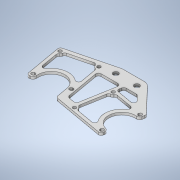
# Autodesk Inventor part: Knee_side_frame
Saved by Autodesk Inventor 2020.4 (Build 244396000, 396)
## iProperties
Created: 2021-09-05
Part Number: Knee_side_frame
Material: アルミニウム 2014-T4
Document SubType Name: Modeling
Designer: Masato Kubotera
Density: 2.8 g/cm^3
Appearance: 滑らか - 淡い灰色
Mass: 7.94371 g
Surface Area: 42.7962 cm^2
Volume: 2.83704 cm^3
Description: A2017 T2
Author: Masato Kubotera
Autodesk Inventor part; units mm, degrees
ref_plane "YZ Plane" through (0, 0, 0) normal (1, 0, 0) x (0, 1, 0)
ref_plane "XZ Plane" through (0, 0, 0) normal (0, 1, 0) x (-1, 0, 0)
ref_plane "XY Plane" through (0, 0, 0) normal (0, 0, 1) x (1, 0, 0)
sketch "スケッチ1" plane through (0, 0, 0) normal (0, 0, 1) x (1, 0, 0)
  line L0 (-46.5961, 42.1731) -> (-4.2493, 49.64) construction
  line L1 (-4.2493, 49.64) -> (1.3074, 18.1262) construction
  line L2 (1.3074, 18.1262) -> (-41.0393, 10.6593) construction
  line L3 (-41.0393, 10.6593) -> (-46.5961, 42.1731) construction
  line L4 (-46.5961, 42.1731) -> (1.3074, 18.1262) construction
  line L5 (-4.2493, 49.64) -> (-41.0393, 10.6593) construction
  line L6 (-43.8177, 26.4162) -> (-1.471, 33.8831) construction
  line L7 (-6.7696, 46.6571) -> (-33.3594, 41.9686) construction
  line L8 (-33.3594, 41.9686) -> (-28.6709, 15.3787) construction
  line L9 (-28.6709, 15.3787) -> (-2.0811, 20.0672) construction
  line L10 (-2.0811, 20.0672) -> (-6.7696, 46.6571) construction
  line L11 (-6.7696, 46.6571) -> (-28.6709, 15.3787) construction
  line L12 (-33.3594, 41.9686) -> (-2.0811, 20.0672) construction
  circle A0 centre (-32, 28.5) radius 10.5 construction
  line L13 (-20.0645, 44.3128) -> (-15.376, 17.723) construction
  circle A1 centre (-6.7696, 46.6571) radius 1.35
  circle A2 centre (-2.0811, 20.0672) radius 1.35
  arc A3 (-36.1041, 41.4846) -> (-33.0796, 39.1957) centre (-33.3594, 41.9686) ccw
  line L14 (-36.1041, 41.4846) -> (-36.5382, 43.9466)
  circle A4 centre (0, 8.5) radius 2.05
  circle A5 centre (0, 8.5) radius 6 construction
  circle A6 centre (0, 8.5) radius 4.6 construction
  line L15 (-36.5382, 43.9466) -> (-4.2493, 49.64)
  line L16 (-4.2493, 49.64) -> (5.8157, 9.9758)
  arc A7 (6, 8.5) -> (5.8157, 9.9758) centre (0, 8.5) ccw
  circle A8 centre (-32, -28.5) radius 10.5 construction
  line L17 (-31.7738, 42.2481) -> (-9.2317, 46.2229)
  arc A9 (-27.0853, 15.6583) -> (-31.7738, 42.2481) centre (-32, 28.5) ccw
  line L18 (-27.0853, 15.6583) -> (-4.5432, 19.6331)
  line L19 (-5.9851, 44.2833) -> (-0.2802, 21.8012)
  arc A10 (-9.2317, 46.2229) -> (-5.9851, 44.2833) centre (-6.7696, 46.6571) ccw
  arc A11 (-0.2802, 21.8012) -> (-4.5432, 19.6331) centre (-2.0811, 20.0672) ccw
  arc A12 (-32.03, 42.203) -> (-34.6889, 41.7341) centre (-33.3594, 41.9686) ccw
  arc A13 (-34.6021, 41.2417) -> (-31.9431, 41.7106) centre (-33.2726, 41.4761) ccw
  line L20 (-34.6889, 41.7341) -> (-34.6021, 41.2417)
  line L21 (-31.9431, 41.7106) -> (-32.03, 42.203)
  arc A14 (-30.0004, 15.1443) -> (-27.3415, 15.6132) centre (-28.6709, 15.3787) ccw
  arc A15 (-27.4283, 16.1056) -> (-30.0873, 15.6367) centre (-28.7578, 15.8711) ccw
  line L22 (-30.0004, 15.1443) -> (-30.0873, 15.6367)
  line L23 (-27.4283, 16.1056) -> (-27.3415, 15.6132)
  line L24 (-49.8407, -37.5393) -> (-42.3738, 4.8074) construction
  line L25 (-42.3738, 4.8074) -> (-10.86, -0.7493) construction
  line L26 (-10.86, -0.7493) -> (-18.3269, -43.0961) construction
  line L27 (-18.3269, -43.0961) -> (-49.8407, -37.5393) construction
  line L28 (-49.8407, -37.5393) -> (-10.86, -0.7493) construction
  line L29 (-42.3738, 4.8074) -> (-18.3269, -43.0961) construction
  line L30 (-34.0838, -40.3177) -> (-26.6169, 2.029) construction
  line L31 (-18.5314, -29.8594) -> (-13.8429, -3.2696) construction
  line L32 (-13.8429, -3.2696) -> (-40.4328, 1.4189) construction
  line L33 (-40.4328, 1.4189) -> (-45.1213, -25.1709) construction
  line L34 (-45.1213, -25.1709) -> (-18.5314, -29.8594) construction
  line L35 (-18.5314, -29.8594) -> (-40.4328, 1.4189) construction
  line L36 (-13.8429, -3.2696) -> (-45.1213, -25.1709) construction
  circle A16 centre (-40.4328, 1.4189) radius 1.35
  arc A17 (-44.8868, -23.8415) -> (-45.3557, -26.5004) centre (-45.1213, -25.1709) ccw
  line L37 (-44.8868, -23.8415) -> (-44.3944, -23.9283)
  line L38 (-44.8633, -26.5873) -> (-45.3557, -26.5004)
  arc A18 (-44.8633, -26.5873) -> (-44.3944, -23.9283) centre (-44.6289, -25.2578) ccw
  line L39 (-32, -28.5) -> (-32, 28.5) construction
  line L40 (-13.8429, -3.2696) -> (-18.5314, -29.8594) construction
  circle A19 centre (-13.8429, -3.2696) radius 1.35
  arc A20 (-18.7659, -31.1889) -> (-18.297, -28.53) centre (-18.5314, -29.8594) ccw
  line L41 (-18.297, -28.53) -> (-18.7894, -28.4431)
  line L42 (-19.2583, -31.1021) -> (-18.7659, -31.1889)
  arc A21 (-18.7894, -28.4431) -> (-19.2583, -31.1021) centre (-19.0239, -29.7726) ccw
  circle A22 centre (0, -8.5) radius 2.05
  circle A23 centre (0, -8.5) radius 6 construction
  line L43 (0, 8.5) -> (0, -8.5) construction
  arc A24 (-30.1333, 17.9133) -> (-33.0796, 39.1957) centre (-32, 28.5) ccw
  arc A25 (-21.3013, -29.5493) -> (-42.4123, -25.8268) centre (-32, -28.5) ccw
  arc A26 (-20.4814, -20.991) -> (-40.2557, -17.5043) centre (-32, -28.5) ccw
  line L44 (-47.9807, -26.9905) -> (-45.0262, -27.5114)
  arc A27 (-45.0262, -27.5114) -> (-42.4123, -25.8268) centre (-44.6289, -25.2578) ccw
  arc A28 (-21.3013, -29.5493) -> (-19.4212, -32.0263) centre (-19.0239, -29.7726) ccw
  line L45 (-16.4668, -32.5472) -> (4.1466, -12.8365)
  line L46 (6, -8.5) -> (6, 8.5)
  arc A29 (4.1466, -12.8365) -> (6, -8.5) centre (0, -8.5) ccw
  line L47 (-14.8529, -23.3942) -> (-6, -14.929)
  arc A30 (-40.8669, -1.0432) -> (-37.9337, 1.4859) centre (-40.4328, 1.4189) ccw
  line L48 (-43.4262, -15.5576) -> (-40.8669, -1.0432)
  line L49 (-37.9337, 1.4859) -> (-16.1684, -2.3519)
  arc A31 (-16.1684, -2.3519) -> (-14.2771, -5.7317) centre (-13.8429, -3.2696) ccw
  line L50 (-16.8364, -20.2461) -> (-14.2771, -5.7317)
  line L51 (-11.3809, -3.7038) -> (-14.8529, -23.3942)
  circle A32 centre (-13.8429, -3.2696) radius 2.4 construction
  arc A33 (-41.98, 15.994) -> (-29.2216, 12.7431) centre (-32, 28.5) ccw construction
  line L52 (-40.7981, 4.5296) -> (-39.3221, 12.9004) construction
  line L53 (-39.3221, 12.9004) -> (-10.9597, 7.8994) construction
  line L54 (-12.4357, -0.4715) -> (-10.9597, 7.8994) construction
  line L55 (-19.4212, -32.0263) -> (-16.4668, -32.5472)
  line L56 (-47.9807, -26.9905) -> (-40.3815, 16.1063)
  line L57 (-40.3815, 16.1063) -> (-30.1333, 17.9133)
  arc A34 (-11.3809, -3.7038) -> (-11.3438, -3.2026) centre (-13.8429, -3.2696) ccw
  line L58 (-11.3438, -3.2026) -> (-6, -4.1448)
  line L59 (-35.5876, 11.6206) -> (-36.9574, 3.8523)
  line L60 (-36.9574, 3.8523) -> (-6, -1.6063)
  line L61 (-6, -1.6063) -> (-6, 16.8377)
  line L62 (-35.5876, 11.6206) -> (-6, 16.8377)
  arc A35 (-43.4262, -15.5576) -> (-40.2557, -17.5043) centre (-41.4566, -15.9049) ccw
  arc A36 (-20.4814, -20.991) -> (-16.8364, -20.2461) centre (-18.806, -19.8988) ccw
  line L63 (-6, -4.1448) -> (-6, -14.929)
  point P0 (-22.6443, 30.1497)
  point P1 (-17.7203, 31.0179)
  point P2 (-30.3503, -19.1443)
  point P3 (-29.4821, -14.2203)
  point P4 (-29.4821, -14.2203)
  point P5 (-44.8417, -23.5853)
  point P6 (-18.2519, -28.2738)
  point P7 (31.7198, -6.6988)
  point P8 (-13.0711, -52.3219)
  point P9 (-12.9341, -52.334)
  point P10 (13.7499, -57.0391)
  point P11 (13.8829, -57.0746)
  point P12 (0, 0)
  point P13 (0, 0)
  dimension "d21" = 43
  dimension "d22" = 32
  dimension "d23" = 27
  dimension "d24" = 27
  dimension "d27" = 21
  dimension "d28" = 9.5
  dimension "d31" = 4.1
  dimension "d34" = 12
  dimension "d39" = 8.5
  dimension "d40" = 9.2
  dimension "d41" = 32
  dimension "d46" = 20
  dimension "d56" = 2.5
  dimension "d57" = 2.5
  dimension "d62" = 3
  dimension "d63" = 2.5
  dimension "d67" = 2.7
  dimension "d68" = 1.35
  dimension "d70" = 0.5
  dimension "d72" = 43
  dimension "d73" = 32
  dimension "d77" = 9.5
  dimension "d78" = 20
  dimension "d80" = 27
  dimension "d81" = 27
  dimension "d82" = 8.5
  dimension "d83" = 2.7
  dimension "d86" = 0.5
  dimension "d87" = 1.35
  dimension "d88" = 57
  dimension "d89" = 80
  dimension "d90" = 21
  dimension "d91" = 100
  dimension "d92" = 4.1
  dimension "d93" = 12
  dimension "d94" = 17
  dimension "d95" = 3
  dimension "d96" = 0.25
  dimension "d97" = 0.25
  dimension "d98" = 3
  dimension "d99" = 0
  dimension "d101" = 2.5
  dimension "d102" = 5.5
  dimension "d107" = 2.5
  dimension "d109" = 2.5
  dimension "d111" = 4.8
  dimension "d112" = 8.5
  dimension "d113" = 28.8
  dimension "d114" = 2.5
  dimension "d115" = 2.5
  dimension "d116" = 2
  dimension "d117" = 2
  dimension "d118" = 2.5
  dimension "d119" = 5.5
  dimension "d120" = 2.5
  constraints: 128 end point, 56 point on circle, 37 centre point, 24 coincident, 23 tangent, 22 parallel, 22 symmetric about line, 16 midpoint, 16 point on line, 11 perpendicular, 3 vertical, 2 collinear, 8 other
  measures "d21" distance of L1.end L2.end
  measures "d22" distance of L0.end L1.end
  measures "d23" distance of L9.end L8.end
  measures "d24" distance of L8.end L7.end
  measures "d27" diameter of A0
  measures "d28" distance of point (-22.644, 30.15) A0.centre
  measures "d31" diameter of A4
  measures "d34" diameter of A5
  measures "d39" distance from line of L8 point (-22.644, 30.15)
  measures "d40" diameter of A6
  measures "d41" horizontal distance of A4.centre A0.centre
  measures "d46" vertical distance of L43.start A0.centre
  measures "d56" radius of A10
  measures "d57" distance from line of L17.end L15
  measures "d62" distance between parallel lines of L16 L19
  measures "d63" radius of A11
  measures "d67" diameter of A1
  measures "d68" radius of A12
  measures "d70" distance of L21.start L21.end
  measures "d72" distance of L25.end L26.end
  measures "d73" distance of L24.end L25.end
  measures "d77" distance of L39.start point (-30.35, -19.144)
  measures "d78" angle of L25 L2
  measures "d80" distance of L31.start L31.end
  measures "d81" distance of L31.end L32.end
  measures "d82" distance from line of L34 point (-30.35, -19.144)
  measures "d83" diameter of A16
  measures "d86" distance of L33.end A18.centre
  measures "d87" radius of A17
  measures "d88" distance of L39.start A0.centre
  measures "d89" angle of L39 L2
  measures "d90" diameter of A8
  measures "d91" angle of L25 L39
  measures "d92" diameter of A22
  measures "d93" diameter of A23
  measures "d94" distance of L43.start L43.end
  measures "d95" radial gap between concentric circles of A24 A9
  measures "d96" radial gap between concentric circles of A0 A24
  measures "d97" radial gap between concentric circles of A8 A25
  measures "d98" radial gap between concentric circles of A25 A26
  measures "d99" distance between parallel lines of L9 L18
  measures "d101" radius of A30
  measures "d102" distance between parallel lines of L45 L47
  measures "d107" distance between parallel lines of L49 L25
  measures "d109" distance between parallel lines of L50 L51
  measures "d111" diameter of A32
  measures "d112" distance of L52.start L52.end
  measures "d113" distance of L52.end L53.end
  measures "d114" distance between parallel lines of L56 L48
  measures "d115" radius of A34
  measures "d116" radius of A35
  measures "d117" radius of A36
  measures "d118" distance between parallel lines of L49 L60
  measures "d119" distance between parallel lines of L56 L59
  measures "d120" distance between parallel lines of L62 L18
extrude "押し出し1" add sketch "スケッチ1" along normal blind 2
fillet "フィレット1" radius 2 6 edges at (-36.5382, 43.9466, 1) (-4.2493, 49.64, 1) (-16.4668, -32.5472, 1) (-47.9807, -26.9905, 1) (-30.1333, 17.9133, 1) (-40.3815, 16.1063, 1)
fillet "フィレット2" radius 2 19 edges at (-31.7738, 42.2481, 1) (-27.0853, 15.6583, 1) (-4.5432, 19.6331, 1) (-9.2317, 46.2229, 1) (-5.9851, 44.2833, 1) (-40.8669, -1.0432, 1) (-14.8529, -23.3942, 1) (-37.9337, 1.4859, 1) (-14.2771, -5.7317, 1) (-16.1684, -2.3519, 1) (-36.9574, 3.8523, 1) (-35.5876, 11.6206, 1) (-11.3438, -3.2026, 1) (-11.3809, -3.7038, 1) (-6, -1.6063, 1) (-6, 16.8377, 1) (-0.2802, 21.8012, 1) (-6, -4.1448, 1) (-6, -14.929, 1)
